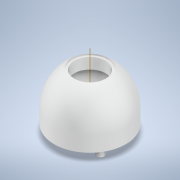
# Autodesk Inventor part: hmm
Saved by Autodesk Inventor 2021 (Build 250183000, 183)
## iProperties
Created: 2020-07-09
Part Number: hmm
Material: Aluminum 6061
Document SubType Name: Modeling
Designer: andre
Density: 2.7 g/cm^3
Appearance: Aluminum - Flat
Author: andre
## iProperties of the stored document _3DPrint.ipt
Created: 2020-07-09
Part Number: _3DPrint
Material: Generic
Document SubType Name: Modeling
Designer: andre
Density: 1 g/cm^3
Appearance: Default
Author: andre
Autodesk Inventor part; units mm, degrees
ref_plane "YZ Plane" through (0, 0, 0) normal (1, 0, 0) x (0, 1, 0)
ref_plane "XZ Plane" through (0, 0, 0) normal (0, 1, 0) x (-1, 0, 0)
ref_plane "XY Plane" through (0, 0, 0) normal (0, 0, 1) x (1, 0, 0)
sketch "Sketch1" plane through (0, 0, 0) normal (0, 1, 0) x (-1, 0, 0)
  line L0 (26, 0) -> (-26, 0)
  line L1 (-26, 0) -> (-26, -26)
  line L2 (-26, -26) -> (26, -26)
  line L3 (26, -26) -> (26, 0)
  point P0 (0, 0)
  dimension "d0" = 52
  dimension "d1" = 26
  dimension "d2" = 26
  dimension "d3" = 26
  constraints: 8 end point, 2 parallel, 1 horizontal, 1 perpendicular
  measures "d0" distance of L2.end L1.end
  measures "d1" distance between parallel lines of L2 L0
  measures "d2" distance from line of point (0, 0) L1
  measures "d3" distance from line of point (0, 0) L2
extrude "Extrusion1" add sketch "Sketch1" along normal blind 35
sketch "Sketch3" plane through (-26, 0, 0) normal (0, 0, 1) x (1, 0, 0)
  line L0 (0, 35) -> (52, 35) projected
  line L1 (38.8, 35) -> (65.2826, 35)
  line L2 (65.2826, 35) -> (65.2826, 0)
  line L3 (26, -13.8937) -> (26, 45.4279) projected
  line L4 (52, 0) -> (52, 35) projected
  arc A0 (52, 10.4979) -> (38.8, 35) centre (22.6594, 10.4979) ccw
  line L5 (52, 10.4979) -> (52, 0)
  line L6 (65.2826, 0) -> (52, 0)
  point P0 (26, 0)
  point P1 (52, 10.9288)
  dimension "d7" = 90
  dimension "d33" = 12.8
  constraints: 8 end point, 2 horizontal, 2 point on circle, 2 point on line, 1 centre point, 1 collinear, 1 tangent
  measures "d7" angle of L1 L2
  measures "d33" horizontal distance of point (26, 0) L1.start
revolve "Revolution1" cut sketch "Sketch3" angle 360 about axis through (0, 35, 0) along (0, 1, 0)
sketch "Sketch2" plane through (0, 35, 0) normal (0, 1, 0) x (1, 0, 0)
  circle A0 centre (0, 0) radius 12.8
  dimension "d6" = 25.6
  constraints: 1 centre point, 1 coincident
  measures "d6" diameter of A0
extrude "Extrusion2" cut sketch "Sketch2" against normal blind 1
sketch "Sketch4" plane through (0, 34, 0) normal (0, 1, 0) x (1, 0, 0)
  circle A0 centre (0, 0) radius 11.4
  dimension "d11" = 22.8
  constraints: 1 centre point, 1 coincident
  measures "d11" diameter of A0
extrude "Extrusion3" cut sketch "Sketch4" against normal through all
sketch "Sketch5" plane through (0, 0, 0) normal (0, -1, 0) x (1, 0, 0)
  circle A0 centre (0, 0) radius 16.4
  dimension "d16" = 32.8
  constraints: 1 centre point, 1 coincident
  measures "d16" diameter of A0
extrude "Extrusion4" cut sketch "Sketch5" against normal blind 26
sketch "Sketch8" plane through (0, 0, 0) normal (0, -1, 0) x (1, 0, 0)
  circle A0 centre (0, -21) radius 2.7
  point P0 (0, 0)
  dimension "d21" = 5.4
  dimension "d22" = 21
  constraints: 1 centre point
  measures "d21" diameter of A0
  measures "d22" distance of point (0, 0) A0.centre
extrude "Extrusion5" add sketch "Sketch8" along normal blind 5
pattern_circular "Circular Pattern1" count 5 over 240 about axis through (0, 35, 0) along (0, 1, 0) of "Extrusion5" both ways yes
mirror "Mirror1" about plane through (-26, 0, 0) normal (0, 0, 1) of "Extrusion4", "Extrusion1", "Revolution1", "Extrusion2", "Extrusion3"
fillet "Fillet2" radius 1 1 edges at (-16.4, 26, 0) curvature continuous yes
equation "\"d1\" = 0.5 * d0"
equation "\"d2\" = 0.5 * d0"
equation "\"d3\" = d1"
equation "\"d33\" = 0.5 * d6"
body "Solid1"
